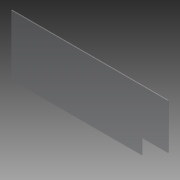
# Autodesk Inventor part: Robot Side
Saved by Autodesk Inventor 2014 (Build 180170000, 170)
## iProperties
Created: 2014-01-23
Part Number: Robot Side
Material: Polycarbonate, Clear
Document SubType Name: Modeling
Designer: Andrew Toennies
Mass: 409.021 g
Surface Area: 2193.54 cm^2
Volume: 340.851 cm^3
Density: 1.2 g/cm^3
Appearance: Polycarbonate - Clear
Author: Andrew Toennies
Autodesk Inventor part; units mm, degrees
ref_plane "YZ Plane" through (0, 0, 0) normal (1, 0, 0) x (0, 1, 0)
ref_plane "XZ Plane" through (0, 0, 0) normal (0, 1, 0) x (-1, 0, 0)
ref_plane "XY Plane" through (0, 0, 0) normal (0, 0, 1) x (1, 0, 0)
sketch "Sketch1" plane through (0, 0, 0) normal (0, 0, 1) x (1, 0, 0)
  line L0 (0, 0) -> (411.6011, 0)
  line L1 (528.32, 50.8) -> (528.32, 203.2)
  line L2 (528.32, 203.2) -> (0, 203.2)
  line L3 (0, 203.2) -> (0, 0)
  line L4 (426.72, 9.525) -> (426.72, 50.8)
  line L5 (426.72, 50.8) -> (528.32, 50.8)
  line L6 (426.72, 9.525) -> (458.47, 9.525)
  line L7 (458.47, 9.525) -> (458.47, 0)
  line L8 (458.47, 0) -> (411.6011, 0)
  dimension "d0" = 528.32
  dimension "d1" = 203.2
  dimension "d5" = 101.6
  dimension "d6" = 31.75
  dimension "d7" = 9.525
  dimension "d8" = 50.8
  constraints: 18 end point, 4 parallel, 4 perpendicular, 1 horizontal
  measures "d0" distance of L1.end L2.end
  measures "d1" distance of L2.end L0.start
  measures "d5" distance of L1.start L4.end
  measures "d6" distance of L4.start L6.end
  measures "d7" distance between parallel lines of L8 L6
  measures "d8" distance between parallel lines of L0 L5
extrude "Extrusion1" add sketch "Sketch1" along normal blind 3.175
body "Solid1"
